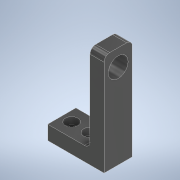
# Autodesk Inventor part: induction_adapter
Saved by Autodesk Inventor 2021 (Build 250183000, 183)
## iProperties
Created: 2022-06-30
Part Number: induction_adapter
Material: ABS Plastic
Document SubType Name: Modeling
Designer: lenna
Density: 1.06 g/cm^3
Appearance: Dark Gray
Author: lenna
Autodesk Inventor part; units mm, degrees
ref_plane "YZ Plane" through (0, 0, 0) normal (1, 0, 0) x (0, 1, 0)
ref_plane "XZ Plane" through (0, 0, 0) normal (0, 1, 0) x (-1, 0, 0)
ref_plane "XY Plane" through (0, 0, 0) normal (0, 0, 1) x (1, 0, 0)
sketch "Sketch1" plane through (0, 0, 0) normal (0, 0, 1) x (1, 0, 0)
  line L0 (0, 72) -> (-10, 72)
  line L1 (-10, 72) -> (-10, 10)
  line L2 (-10, 10) -> (-40, 10)
  line L3 (-40, 10) -> (-40, 0)
  line L4 (-40, 0) -> (0, 0)
  line L5 (0, 0) -> (0, 72)
  dimension "d0" = 10
  dimension "d1" = 40
  dimension "d2" = 10
  dimension "d3" = 72
  constraints: 12 end point, 5 perpendicular, 1 horizontal
  measures "d0" distance between parallel lines of L4 L2
  measures "d1" distance between parallel lines of L5 L3
  measures "d2" distance between parallel lines of L5 L1
  measures "d3" distance between parallel lines of L4 L0
extrude "Extrusion1" add sketch "Sketch1" along normal mid plane 20
sketch "Sketch2" plane through (0, 0, 10) normal (1, 0, 0) x (0, 0, -1)
  circle A0 centre (10, 60) radius 7
  line L0 (20, 72) -> (0, 72) projected
  point P0 (10, 0)
  dimension "d6" = 0
  dimension "d7" = 12
  dimension "d8" = 14
  constraints: 1 centre point
  measures "d6" horizontal distance of point (10, 0) A0.centre
  measures "d7" distance from line of L0 A0.centre
  measures "d8" diameter of A0
extrude "Extrusion2" cut sketch "Sketch2" against normal up to surface (10 mm away)
fillet "Fillet1" radius 4 3 edges at (-5, 72, 10) (-5, 72, -10) (-10, 10, 0)
sketch "Sketch3" plane through (-40, 10, 10) normal (0, 1, 0) x (1, 0, 0)
  line L0 (26, 0) -> (0, 0) projected
  line L1 (0, 20) -> (26, 20) projected
  line L2 (0, 20) -> (0, 0) projected
  point P0 (40, 10)
  point P1 (7, 10)
  point P2 (20, 10)
  dimension "d19" = 20
  dimension "d20" = 10
  dimension "d21" = 0
  dimension "d22" = 7
  dimension "d23" = 13
  measures "d19" distance between parallel lines of L0 L1
  measures "d20" distance from line of L1 point (7, 10)
  measures "d21" vertical distance of point (20, 10) point (7, 10)
  measures "d22" distance from line of L2 point (7, 10)
  measures "d23" distance of point (7, 10) point (20, 10)
hole "Hole1" at (-33, 10, 0) at (-20, 10, 0) direction (0, -1, 0) diameter 5.5 depth 10 counterbore diameter 9 counterbore depth 5
equation "\"d20\" = 0.5 * d19"
body "Solid1"
